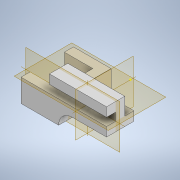
# Autodesk Inventor part: Hanging_Wall
Saved by Autodesk Inventor 2022.4 (Build 264492010, 492A)
## iProperties
Created: 2025-02-20
Part Number: Hanging_Wall
Material: Generic
Document SubType Name: Modeling
Designer: jan-m
Density: 1 g/cm^3
Appearance: Default
Author: jan-m
Autodesk Inventor part; units mm, degrees
sketch "Sketch2" plane through (0, 0, 0) normal (1, 0, 0) x (0, 1, 0)
  line L0 (0, -7.6) -> (0, -1.6)
  line L1 (0, 3.44) -> (0, -9.44) projected
  line L2 (-5.4, 0) -> (4.4, 0) projected
  line L3 (0, -1.6) -> (3, -1.6)
  line L4 (3, -1.6) -> (3, 1.6)
  line L5 (3, 1.6) -> (1.4, 1.6)
  line L6 (1.4, 1.6) -> (1.4, 0)
  line L7 (1.4, 0) -> (0, 0)
  line L8 (0, 0) -> (0, 1.6)
  line L9 (0, 1.6) -> (-4, 1.6)
  line L10 (-4, 1.6) -> (-4, 1.6)
  line L11 (-4, 1.6) -> (-4, -7.6)
  line L12 (-4, -7.6) -> (0, -7.6)
  point P0 (0, 0)
  dimension "d1" = 6
  dimension "d2" = 3
  dimension "d3" = 3.2
  dimension "d4" = 1.6
  dimension "d6" = 4
  dimension "d7" = 1.6
  dimension "d8" = 1.4
  dimension "d12" = 1.6
  constraints: 22 end point, 6 perpendicular, 2 horizontal, 1 vertical
  measures "d1" distance of L0.start L0.end
  measures "d2" distance of L0.end L3.end
  measures "d3" distance of L3.end L4.end
  measures "d4" distance of L4.end L5.end
  measures "d6" distance of L8.end L9.end
  measures "d7" distance of L7.end L8.end
  measures "d8" distance between parallel lines of L6 L8
  measures "d12" distance between parallel lines of L3 L7
extrude "Extrusion1" add sketch "Sketch2" along normal mid plane 10
sketch "Sketch3" plane through (0, 0, 0) normal (0, 0, 1) x (1, 0, 0)
  line L0 (5, 0) -> (5, 3) projected
  line L1 (5, 0) -> (5, -1.6)
  line L2 (5, -4) -> (5, 0) projected
  line L3 (-5, -4) -> (5, -4) projected
  line L4 (-3.4, -4) -> (-3.4, -4)
  line L5 (-5, 0) -> (-5, -4) projected
  line L6 (5, -1.6) -> (-1, -1.6)
  arc A0 (-1, -1.6) -> (-3.4, -4) centre (-1, -4) ccw
  point P0 (0, 0)
  point P1 (-3.4, -4)
  dimension "d14" = 1.6
  dimension "d15" = 1.6
  dimension "d17" = 2.4
  constraints: 6 end point, 2 point on circle, 2 point on line, 2 tangent, 1 centre point, 1 perpendicular, 1 vertical
  measures "d14" distance of L0.start L1.end
  measures "d15" distance between parallel lines of L5 L4
  measures "d17" radius of A0
extrude "Extrusion2" cut sketch "Sketch3" along normal through all both and the other way through all
sketch "Sketch4" plane through (-5, 0, 0) normal (-1, 0, 0) x (0, 0, 1)
  line L0 (1.6, 0) -> (0, 0) projected
  line L1 (-7.6, -4) -> (1.6, -4) projected
  line L2 (1.6, 0) -> (0, 0)
  line L3 (0, 0) -> (0, -4)
  line L4 (0, -4) -> (1.6, -4)
  line L5 (1.6, -4) -> (1.6, 0)
  line L6 (-1.6, 0) -> (-7.6, 0) projected
  line L7 (-7.6, 0) -> (-6, 0)
  line L8 (-6, 0) -> (-6, -4)
  line L9 (-6, -4) -> (-7.6, -4)
  line L10 (-7.6, -4) -> (-7.6, 0)
  point P0 (1.6, -4)
  dimension "d20" = 1.6
  dimension "d21" = 1.6
  constraints: 16 end point, 4 parallel, 2 horizontal, 2 perpendicular, 2 point on line
  measures "d20" distance between parallel lines of L5 L3
  measures "d21" distance of L8.end L9.end
sketch "Sketch5" plane through (5, 0, -7.6) normal (0, 0, -1) x (-1, 0, 0)
  point P0 (5, 0)
extrude "Extrusion3" add sketch "Sketch4" along normal blind 5
sketch "Sketch6" plane through (-5, 0, -1.6) normal (0, 1, 0) x (1, 0, 0)
  line L0 (-5, 6) -> (10, 6) projected
  line L1 (1.6, 6) -> (1.6, 3.2)
  line L2 (0, 0) -> (0, 4.4) projected
  line L3 (10, 6) -> (10, 0) projected
  line L4 (10, 1.6) -> (3.2, 1.6)
  line L5 (0, 0) -> (10, 0) projected
  arc A0 (1.6, 3.2) -> (3.2, 1.6) centre (3.2, 3.2) ccw
  point P0 (5, -1.6)
  dimension "d24" = 1.6
  dimension "d25" = 1.6
  dimension "d26" = 1.6
  constraints: 4 end point, 2 point on circle, 2 point on line, 2 tangent, 1 centre point, 1 horizontal, 1 vertical
  measures "d24" distance between parallel lines of L1 L2
  measures "d25" distance between parallel lines of L5 L4
  measures "d26" radius of A0
extrude "Extrusion4" cut sketch "Sketch6" along normal through all both and the other way through all
body "Solid1"
